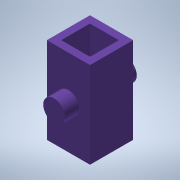
# Autodesk Inventor part: SlderA
Saved by Autodesk Inventor 2021 (Build 250183000, 183)
## iProperties
Created: 2015-03-05
Part Number: SlderA
Document SubType Name: Modeling
Designer: Administrator
Density: 1 g/cm^3
Mass: 0.0335343 g
Surface Area: 1.39425 cm^2
Volume: 0.0335343 cm^3
Material: Generic
Appearance: Violet
Author: Administrator
Autodesk Inventor part; units mm, degrees
ref_plane "YZ Plane" through (0, 0, 0) normal (1, 0, 0) x (0, 1, 0)
ref_plane "XZ Plane" through (0, 0, 0) normal (0, 1, 0) x (-1, 0, 0)
ref_plane "XY Plane" through (0, 0, 0) normal (0, 0, 1) x (1, 0, 0)
sketch "Sketch9" plane through (0, 0, 0) normal (0, 0, 1) x (1, 0, 0)
  line L0 (1, 1) -> (1, -1)
  line L1 (1, -1) -> (-1, -1)
  line L2 (-1, -1) -> (-1, 1)
  line L3 (-1, 1) -> (1, 1)
  line L4 (-1.5, 1.5) -> (-1.5, -1.5)
  line L5 (-1.5, -1.5) -> (1.5, -1.5)
  line L6 (1.5, -1.5) -> (1.5, 1.5)
  line L7 (1.5, 1.5) -> (-1.5, 1.5)
  point P0 (0, 0)
  dimension "d36" = 2
  dimension "d37" = 3
  constraints: 16 end point, 13 other
  measures "d36" distance of L2.end L0.start
  measures "d37" distance of L6.end L4.start
extrude "Extrusion7" add sketch "Sketch9" along normal mid plane 6
sketch "Sketch10" plane through (0, 0, 0) normal (0, 0, 1) x (1, 0, 0)
  line L0 (-1.5, 1.5) -> (1.5, 1.5) projected
  line L1 (1.5, -1.5) -> (-1.5, -1.5) projected
  line L2 (0, 1.5) -> (0, -1.5) construction
  line L3 (0, 1.5) -> (-0.75, 1.5)
  line L4 (-0.75, 1.5) -> (-0.75, 2.5)
  line L5 (-0.75, 2.5) -> (0, 2.5)
  line L6 (0, 2.5) -> (0, 1.5)
  line L7 (0, -1.5) -> (-0.75, -1.5)
  line L8 (-0.75, -1.5) -> (-0.75, -2.5)
  line L9 (-0.75, -2.5) -> (0, -2.5)
  line L10 (0, -2.5) -> (0, -1.5)
  dimension "d40" = 0.75
  dimension "d42" = 1
  dimension "d43" = 1
  constraints: 18 end point, 5 parallel, 2 horizontal, 2 midpoint, 2 perpendicular
  measures "d40" distance of L4.end L5.end
  measures "d42" distance of L5.end L2.start
  measures "d43" distance of L9.end L2.end
revolve "Revolution2" add sketch "Sketch10" angle 360 about axis through (0, 1.5, 0) along (0, -1, 0)
body "Solid1"
